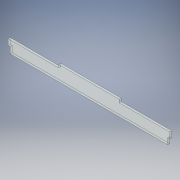
# Autodesk Inventor part: Refuerzo_Base
Saved by Autodesk Inventor 2019 (Build 230136000, 136)
## iProperties
Created: 2020-04-07
Part Number: Refuerzo_Base
Material: Generic
Document SubType Name: Modeling
Designer: Jurgen
Density: 1 g/cm^3
Appearance: Clear
Author: Jurgen
Autodesk Inventor part; units mm, degrees
ref_plane "YZ Plane" through (0, 0, 0) normal (1, 0, 0) x (0, 1, 0)
ref_plane "XZ Plane" through (0, 0, 0) normal (0, 1, 0) x (-1, 0, 0)
ref_plane "XY Plane" through (0, 0, 0) normal (0, 0, 1) x (1, 0, 0)
sketch "Sketch1" plane through (0, 0, 0) normal (0, 0, 1) x (1, 0, 0)
  line L0 (0, 0) -> (-267, 0)
  line L1 (-267, 0) -> (-267, 10)
  line L2 (-267, 10) -> (-263.5, 10)
  line L3 (-263.5, 10) -> (-263.5, 20)
  line L4 (-3.5, 20) -> (-3.5, 10)
  line L5 (-3.5, 10) -> (0, 10)
  line L6 (0, 10) -> (0, 0)
  line L7 (-83.5, 20) -> (-83.5, 25)
  line L8 (-83.5, 25) -> (-183.5, 25)
  line L9 (-183.5, 25) -> (-183.5, 20)
  line L10 (-263.5, 20) -> (-183.5, 20)
  line L11 (-83.5, 20) -> (-3.5, 20)
  dimension "d19" = 267
  dimension "d20" = 10
  dimension "d22" = 10
  dimension "d23" = 260
  dimension "d24" = 100
  dimension "d25" = 5
  dimension "d26" = 80
  constraints: 24 end point, 8 perpendicular, 2 point on line, 1 horizontal, 1 parallel
  measures "d19" distance of L0.start L0.end
  measures "d20" distance of L0.end L1.end
  measures "d22" distance of L2.end L3.end
  measures "d23" distance of L3.end L4.start
  measures "d24" distance of L8.end L7.end
  measures "d25" distance of L7.end L7.start
  measures "d26" distance between parallel lines of L4 L7
extrude "Extrusion1" add sketch "Sketch1" along normal blind 3.5
sketch "Sketch2" plane through (0, 0, 3.5) normal (0, 0, 1) x (1, 0, 0)
  line L0 (-267, 0) -> (0, 0) construction
  line L1 (0, 0) -> (0, 10) construction
  line L2 (0, 10) -> (-3.5, 10) projected
  line L3 (-3.5, 10) -> (-3.5, 20) projected
  line L4 (-3.5, 20) -> (-83.5, 20) construction
  line L5 (-83.5, 20) -> (-83.5, 25) construction
  line L6 (-83.5, 25) -> (-183.5, 25) construction
  line L7 (-183.5, 25) -> (-183.5, 20) construction
  line L8 (-183.5, 20) -> (-263.5, 20) construction
  line L9 (-263.5, 20) -> (-263.5, 10) projected
  line L10 (-263.5, 10) -> (-267, 10) projected
  line L11 (-267, 10) -> (-267, 0) construction
  line L12 (-263.5, 10) -> (-267, 10)
  line L13 (-267, 10) -> (-267, 20)
  line L14 (-267, 20) -> (-263.5, 20)
  line L15 (-263.5, 20) -> (-263.5, 10)
  line L16 (-3.5, 10) -> (0, 10)
  line L17 (0, 10) -> (0, 20)
  line L18 (0, 20) -> (-3.5, 20)
  line L19 (-3.5, 20) -> (-3.5, 10)
  constraints: 16 end point, 4 parallel, 2 horizontal, 2 perpendicular
extrude "Extrusion2" add sketch "Sketch2" against normal blind 3.5
sketch "Sketch3" plane through (0, 0, 3.5) normal (0, 0, 1) x (1, 0, 0)
  line L0 (-267, 0) -> (0, 0) construction
  line L1 (0, 0) -> (0, 20) construction
  line L2 (0, 20) -> (-83.5, 20) construction
  line L3 (-83.5, 20) -> (-83.5, 25) construction
  line L4 (-83.5, 25) -> (-183.5, 25) construction
  line L5 (-183.5, 25) -> (-183.5, 20) construction
  line L6 (-183.5, 20) -> (-267, 20) construction
  line L7 (-267, 0) -> (-267, 20) construction
  line L8 (-267, 0) -> (-267, 20) projected
  line L9 (-267, 0) -> (-263.5, 0)
  line L10 (-263.5, 0) -> (-263.5, 10)
  line L11 (-263.5, 10) -> (-267, 10)
  line L12 (-267, 10) -> (-267, 0)
  line L13 (0, 0) -> (-3.5, 0)
  line L14 (-3.5, 0) -> (-3.5, 10)
  line L15 (-3.5, 10) -> (0, 10)
  line L16 (0, 10) -> (0, 0)
  dimension "d29" = 3.5
  dimension "d30" = 10
  dimension "d31" = 3.5
  dimension "d32" = 10
  constraints: 16 end point, 4 parallel, 2 horizontal, 2 perpendicular
  measures "d29" distance of L11.end L10.end
  measures "d30" distance of L10.end L9.end
  measures "d31" distance of L14.end L15.end
  measures "d32" distance of L13.end L14.end
extrude "Extrusion3" cut sketch "Sketch3" against normal blind 3.5
body "Solid1"
